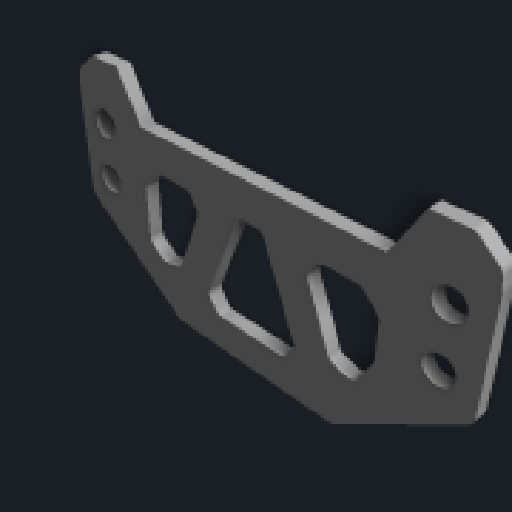
# Autodesk Inventor part: NoseMount
Saved by Autodesk Inventor 2025.2 (Build 292293000, 293)
## iProperties
Created: 2024-12-21
Part Number: NoseMount
Material: Generic
Document SubType Name: Sheet Metal
Designer: valer
Density: 1 g/cm^3
Sheet Metal Rule: Default
Appearance: Default
Author: valer
Autodesk Inventor part; units mm, degrees
ref_plane "YZ Plane" through (0, 0, 0) normal (1, 0, 0) x (0, 1, 0)
ref_plane "XZ Plane" through (0, 0, 0) normal (0, 1, 0) x (-1, 0, 0)
ref_plane "XY Plane" through (0, 0, 0) normal (0, 0, 1) x (1, 0, 0)
sketch "Sketch1" plane through (0, 0, 0) normal (0, 0, 1) x (1, 0, 0)
  circle A0 centre (11, 6) radius 2.7 construction
  circle A1 centre (11, -6) radius 2.7 construction
  line L0 (49.7615, -342.4426) -> (49.7615, 314.6303) construction
  line L1 (11, 12) -> (-4.4335, 12) construction
  line L2 (-17, -12) -> (11, -12) construction
  line L3 (4, 12) -> (4, -12)
  line L4 (4, 12) -> (5.1669, 19)
  line L5 (5.1669, 19) -> (49.7615, 19)
  line L6 (5.1669, 19) -> (26.8834, 2.9834) construction
  line L7 (19.0192, 2.5843) -> (28.2364, 13.6384) construction
  circle A2 centre (11, 6) radius 3
  circle A3 centre (11, -6) radius 3
  circle A4 centre (88.5231, 6) radius 3
  circle A5 centre (88.5231, -6) radius 3
  line L8 (4, -12) -> (29.7615, -31)
  line L9 (29.7615, -31) -> (49.7615, -31)
  line L10 (95.5231, 12) -> (95.5231, -12)
  line L11 (95.5231, 12) -> (94.3561, 19)
  line L12 (94.3561, 19) -> (49.7615, 19)
  line L13 (95.5231, -12) -> (69.7615, -31)
  line L14 (69.7615, -31) -> (49.7615, -31)
  point P0 (0, 0)
  dimension "d0" = 7
  dimension "d6" = 6
  dimension "d7" = 6
  dimension "d8" = 7
  dimension "d14" = 7
  dimension "d15" = 50
  dimension "d16" = 20
  measures "d0" distance from line of A0.centre L3
  measures "d6" diameter of A2
  measures "d7" diameter of A3
  measures "d8" distance from line of L6 A0.centre
  measures "d14" distance between parallel lines of L5 L1
  measures "d15" distance between parallel lines of L9 L5
  measures "d16" distance of L8.end L9.end
extrude "Plate1" add sketch "Sketch1" along normal blind 3.048
sketch "Sketch2" plane through (0, 0, 3.048) normal (0, 0, 1) x (1, 0, 0)
  line L0 (4, -12) -> (29.7615, -31) construction
  line L1 (49.7615, 19) -> (29.7615, -31) construction
  line L2 (29.7615, -31) -> (69.7615, -31) construction
  line L3 (49.7615, 19) -> (69.7615, -31) construction
  line L4 (5.1669, 19) -> (94.3561, 19) construction
  line L5 (35.6697, -27) -> (49.7615, 8.2297)
  line L6 (49.7615, 8.2297) -> (63.8534, -27)
  line L7 (63.8534, -27) -> (35.6697, -27)
  line L8 (38.3453, 1.2297) -> (29.5052, -20.8705)
  line L9 (29.5052, -20.8705) -> (22.1239, -15.4265)
  line L10 (22.1239, -15.4265) -> (22.1239, 1.2297)
  line L11 (22.1239, 1.2297) -> (38.3453, 1.2297)
  line L12 (4, -12) -> (4, 12) projected
  line L13 (37.2697, -23) -> (62.2534, -23)
  line L14 (49.7615, 19) -> (49.7615, -31) construction
  line L15 (61.1778, 1.2297) -> (70.0179, -20.8705)
  line L16 (70.0179, -20.8705) -> (77.3992, -15.4265)
  line L17 (77.3992, -15.4265) -> (77.3992, 1.2297)
  line L18 (77.3992, 1.2297) -> (61.1778, 1.2297)
  line L19 (16.483, 19) -> (22.1239, 9.2297)
  line L20 (22.1239, 9.2297) -> (49.7615, 9.2297)
  line L21 (22.1239, 9.2297) -> (22.1239, 1.2297) construction
  line L22 (83.0401, 19) -> (77.3992, 9.2297)
  line L23 (77.3992, 9.2297) -> (49.7615, 9.2297)
  line L24 (16.483, 19) -> (83.0401, 19)
  line L25 (94.3561, 19) -> (5.1669, 19) projected
  point P0 (0, 0)
  dimension "d17" = 4
  dimension "d19" = 8
  dimension "d21" = 4
  dimension "d22" = 8
  dimension "d29" = 60
  dimension "d30" = 8
  dimension "d31" = 1
  constraints: 42 end point, 6 symmetric about line, 4 parallel, 4 point on line, 2 midpoint, 2 vertical, 1 collinear, 1 horizontal, 1 perpendicular, 2 other
  measures "d17" distance between parallel lines of L1 L5
  measures "d19" distance between parallel lines of L0 L9
  measures "d21" distance between parallel lines of L1 L8
  measures "d22" distance between parallel lines of L2 L13
  measures "d29" angle of L4 L19
  measures "d30" distance between parallel lines of L11 L20
  measures "d31" distance from line of L23 L5.end
extrude "Cut1" cut sketch "Sketch2" against normal blind 3.048 contours L5 L6 L13 | L8 L9 L10 L11 | L18 L17 L16 L15 | L24 L22 L23 L20 L19
chamfer "Chamfer2" distance 4 angle 45 11 edges at (5.1669, 19, 1.524) (94.3561, 19, 1.524) (29.5052, -20.8705, 1.524) (22.1239, 1.2297, 1.524) (38.3453, 1.2297, 1.524) (37.2697, -23, 1.524) (62.2534, -23, 1.524) (77.3992, -15.4265, 1.524) (70.0179, -20.8705, 1.524) (61.1778, 1.2297, 1.524) (77.3992, 1.2297, 1.524)
fillet "Fillet1" radius 2 29 edges at (26.1239, 1.2297, 1.524) (22.1239, -2.7703, 1.524) (22.1239, -15.4265, 1.524) (26.2861, -18.4962, 1.524) (34.3453, 1.2297, 1.524) (36.8597, -2.4842, 1.524) (30.9908, -17.1566, 1.524) (38.7552, -19.2861, 1.524) (41.2697, -23, 1.524) (58.2534, -23, 1.524) (60.7678, -19.2861, 1.524) (74.18, -17.8007, 1.524) (77.3992, -11.4265, 1.524) (77.3992, -2.7703, 1.524) (73.3992, 1.2297, 1.524) (65.1778, 1.2297, 1.524) (62.6634, -2.4842, 1.524) (68.5323, -17.1566, 1.524) (73.237, -18.4962, 1.524) (69.7615, -31, 1.524) (95.5231, -12, 1.524) (95.5231, 12, 1.524) (29.7615, -31, 1.524) (4, -12, 1.524) (4, 12, 1.524) (4.5092, 15.0544, 1.524) (9.1669, 19, 1.524) (90.3561, 19, 1.524) (95.0139, 15.0544, 1.524)
sketch "Sketch3" plane through (0, 0, 3.048) normal (0, 0, 1) x (1, 0, 0)
  line L0 (26.9523, 1.2297) -> (33.2841, 1.2297)
  line L1 (33.2841, 1.2297) -> (66.239, 1.2297)
  line L2 (66.239, 1.2297) -> (49.7615, 9.2297)
  line L3 (22.1239, 9.2297) -> (77.3992, 9.2297)
  line L4 (33.2841, 1.2297) -> (49.7615, 9.2297)
  point P0 (0, 0)
sheet face with bend "Face2" sketch "Sketch3" thickness 3.048 toward (0, 0, -1) bend radius 3.048 relief straight relief width 3.048 relief depth 1.524
bend "Bend1"
fillet "Fillet2" radius 2 6 edges at (46.9615, 1.2297, 1.524) (52.5615, 1.2297, 1.524) (16.483, 19, 1.524) (83.0401, 19, 1.524) (22.1239, 9.2297, 1.524) (77.3992, 9.2297, 1.524)
equation "\"d19\" = 2 * d17"
equation "\"d21\" = d17"
equation "\"d22\" = 2 * d17"
equation "\"d23\" = Thickness"
equation "\"d9\" = Thickness"
equation "\"BendRadius\" = Thickness"
equation "\"BendReliefWidth\" = Thickness"
equation "\"BendReliefDepth\" = 0.5 * Thickness"
equation "\"CornerReliefSize\" = 4 * Thickness"
equation "\"MinimumRemnant\" = 2 * Thickness"
equation "\"TransitionRadius\" = BendRadius"
equation "\"JacobiRadiusSize\" = BendRadius"
equation "\"GapSize\" = Thickness"
equation "\"Thickness\" = 3.048"
body "Solid1"
